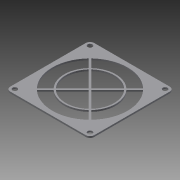
# Autodesk Inventor part: grid
Saved by Autodesk Inventor 2015 (Build 190159000, 159)
## iProperties
Created: 2014-08-15
Part Number: grid
Material: Generic
Document SubType Name: Modeling
Designer: Christo
Density: 1 g/cm^3
Appearance: Default
Author: Christo
Autodesk Inventor part; units mm, degrees
ref_plane "YZ Plane" through (0, 0, 0) normal (1, 0, 0) x (0, 1, 0)
ref_plane "XZ Plane" through (0, 0, 0) normal (0, 1, 0) x (-1, 0, 0)
ref_plane "XY Plane" through (0, 0, 0) normal (0, 0, 1) x (1, 0, 0)
sketch "Sketch1" plane through (0, 0, 0) normal (0, 0, 1) x (1, 0, 0)
  circle A0 centre (-35.75, 35.75) radius 2.25 projected
  circle A1 centre (35.75, 35.75) radius 2.25 projected
  circle A2 centre (35.75, -35.75) radius 2.25 projected
  circle A3 centre (-35.75, -35.75) radius 2.25 projected
  line L0 (40, 40) -> (-40, 40) projected
  line L1 (-40, 40) -> (-40, -40) projected
  line L2 (-40, -40) -> (40, -40) projected
  line L3 (40, -40) -> (40, 40) projected
  circle A4 centre (0, 0) radius 35.75 construction
  line L4 (-35.75, 35.75) -> (35.75, -35.75) construction
  line L5 (-35.75, -35.75) -> (35.75, 35.75) construction
  line L6 (-24.5621, 25.9763) -> (-16.5896, 18.0038) construction
  line L7 (-25.9763, 24.5621) -> (16.5896, -18.0038) construction
  line L8 (24.5621, 25.9763) -> (18.5727, 19.987) construction
  line L9 (-24.5621, -25.9763) -> (16.9422, 15.528) construction
  line L10 (18.5727, 19.987) -> (17.1575, 18.5717) construction
  line L11 (17.1575, 18.5717) -> (16.5896, 18.0038) construction
  line L12 (0, 1.4142) -> (-18.0038, -16.5896) construction
  line L13 (0, 1.4142) -> (16.9422, -15.528) construction
  line L14 (16.5896, 18.0038) -> (15.528, 16.9422) construction
  line L15 (15.528, 16.9422) -> (0, 1.4142) construction
  arc A5 (16.9422, -15.528) -> (16.9422, 15.528) centre (0, 0) ccw
  line L16 (18.0038, 16.5896) -> (25.9763, 24.5621) construction
  line L17 (-16.5896, 18.0038) -> (0, 1.4142) construction
  arc A6 (-16.9422, 15.528) -> (-16.9422, -15.528) centre (0, 0) ccw
  arc A7 (-18.0038, 16.5896) -> (-18.0038, -16.5896) centre (0, 0) ccw
  line L18 (-18.0038, -16.5896) -> (-25.9763, -24.5621) construction
  arc A8 (-16.5896, -18.0038) -> (16.5896, -18.0038) centre (0, 0) ccw
  arc A9 (-15.528, -16.9422) -> (15.528, -16.9422) centre (0, 0) ccw
  line L19 (18.0038, -16.5896) -> (25.9763, -24.5621) construction
  line L20 (16.9422, -15.528) -> (18.0038, -16.5896) construction
  line L21 (16.9422, 15.528) -> (18.0038, 16.5896) construction
  arc A10 (15.528, 16.9422) -> (-15.528, 16.9422) centre (0, 0) ccw
  arc A11 (16.5896, 18.0038) -> (-16.5896, 18.0038) centre (0, 0) ccw
  line L22 (16.5896, -18.0038) -> (24.5621, -25.9763) construction
  arc A12 (18.0038, -16.5896) -> (18.0038, 16.5896) centre (0, 0) ccw
  arc A13 (24.5621, 25.9763) -> (-24.5621, 25.9763) centre (0, 0) ccw
  arc A14 (25.9763, -24.5621) -> (25.9763, 24.5621) centre (0, 0) ccw
  arc A15 (-24.5621, -25.9763) -> (24.5621, -25.9763) centre (0, 0) ccw
  arc A16 (-25.9763, 24.5621) -> (-25.9763, -24.5621) centre (0, 0) ccw
  line L23 (-16.5896, 18.0038) -> (-24.5621, 25.9763)
  line L24 (-18.0038, 16.5896) -> (-25.9763, 24.5621)
  line L25 (16.5896, 18.0038) -> (24.5621, 25.9763)
  line L26 (25.9763, 24.5621) -> (18.0038, 16.5896)
  line L27 (18.0038, -16.5896) -> (25.9763, -24.5621)
  line L28 (24.5621, -25.9763) -> (16.5896, -18.0038)
  line L29 (-24.5621, -25.9763) -> (-16.5896, -18.0038)
  line L30 (-18.0038, -16.5896) -> (-25.9763, -24.5621)
  line L31 (-16.9422, -15.528) -> (-1.4142, 0)
  line L32 (-15.528, -16.9422) -> (0, -1.4142)
  line L33 (-1.4142, 0) -> (-16.9422, 15.528)
  line L34 (-15.528, 16.9422) -> (0, 1.4142)
  line L35 (0, -1.4142) -> (15.528, -16.9422)
  line L36 (16.9422, -15.528) -> (1.4142, 0)
  line L37 (1.4142, 0) -> (16.9422, 15.528)
  line L38 (15.528, 16.9422) -> (0, 1.4142)
  dimension "d8" = 2
  dimension "d9" = 1
  constraints: 70 end point, 46 parallel, 29 point on circle, 15 point on line, 12 centre point, 6 coincident, 5 collinear, 2 perpendicular, 9 other
  measures "d8" distance between parallel lines of L6 L7
  measures "d9" distance between parallel lines of L4 L7
extrude "Extrusion3" add sketch "Sketch1" along normal blind 1.5
fillet "Fillet3" radius 4 4 edges at (-40, -40, 0.75) (40, -40, 0.75) (40, 40, 0.75) (-40, 40, 0.75)
body "Solid3"
